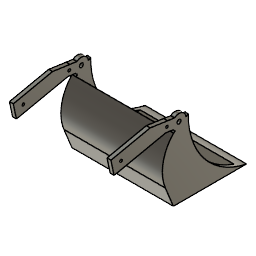
Final Scoop (Autodesk Fusion 360 design; units mm, degrees)
Autodesk Fusion 360 part; units mm, degrees
sketch "Sketch1" plane through (0, 0, 0) normal (1, 0, 0) x (0, 1, 0)
  line L0 (0, 0) -> (254, 0) construction
  line L1 (0, 0) -> (50.8, 0) construction
  line L2 (50.8, 0) -> (50.8, 107.95) construction
  line L3 (50.8, 107.95) -> (117.7014, 0) construction
  line L4 (50.8, 107.95) -> (117.6994, 215.9013) construction
  line L5 (117.7014, 0) -> (212.9514, 0) construction
  line L6 (117.7014, 0) -> (24.5328, 19.8036)
  line L7 (117.7014, 0) -> (212.9514, 0) construction
  line L8 (24.5328, 19.8036) -> (19.6811, 47.3191)
  line L9 (24.5328, 19.8036) -> (52.4728, 19.8036) construction
  arc A0 (41.91, 100.33) -> (19.6811, 47.3191) centre (72.0035, 56.545) ccw
  line L10 (41.91, 100.33) -> (64.77, 100.33) construction
  arc A1 (63.3914, 108.1486) -> (117.7014, 0) centre (155.1008, 86.4922) ccw
  circle A2 centre (50.8, 107.95) radius 2.5654
  line L11 (41.91, 100.33) -> (44.3855, 101.231)
  line L12 (60.0326, 106.9261) -> (63.3914, 108.1486)
  arc A3 (55.3791, 100.33) -> (55.4831, 100.3935) centre (50.8, 107.95) ccw
  line L13 (23.6346, 124.9202) -> (23.6308, 124.9202)
  line L14 (50.8, 107.95) -> (35.8756, 113.3608) construction
  circle A4 centre (35.8756, 113.3608) radius 1.651
  line L15 (46.5903, 116.2306) -> (38.0399, 119.3306)
  arc A5 (60.0326, 106.9261) -> (46.5903, 116.2306) centre (50.8, 107.95) ccw
  arc A6 (42.2617, 104.2911) -> (44.3855, 101.231) centre (50.8, 107.95) ccw
  circle A7 centre (-24.3224, 117.475) radius 1.651
  line L16 (-35.6254, 127.2794) -> (16.51, 127.2794)
  line L17 (38.0399, 119.3306) -> (16.51, 127.2794)
  line L18 (-35.6254, 127.2794) -> (-35.6254, 107.6706)
  line L19 (-35.6254, 107.6706) -> (33.057, 107.6706)
  line L20 (33.057, 107.6706) -> (42.2617, 104.2911)
  point P0 (0, 127)
  point P1 (50.8, 107.95)
  point P2 (-24.3224, 117.475)
  dimension "d1" = 254
  dimension "d2" = 107.95
  dimension "d3" = 127
  dimension "d4" = 127
  dimension "d8" = 95.25
  dimension "d9" = 168
  dimension "d10" = 100
  dimension "d11" = 27.94
  dimension "d14" = 20
  dimension "d15" = 22.86
  dimension "d16" = 5.1308
  dimension "d17" = 17.78
  dimension "d38" = 15.875
  dimension "d40" = 3.302
  dimension "d65" = 3.302
  dimension "d68" = 19.6088
  constraint coincident L0.start L1.start
  constraint horizontal L0
  constraint coincident L0 L1.end
  constraint perpendicular L0 L2
  constraint coincident P1 L2.end
  constraint coincident L0 L3.end
  constraint horizontal L5
  constraint horizontal L7
  constraint horizontal L9
  constraint tangent L8 A0
  constraint horizontal L10
  constraint collinear L11 L12
  constraint coincident L10 A3.start
  constraint coincident L3 A3.end
  constraint concentric A3 A5
  constraint horizontal L13
  constraint concentric A5 A6
  constraint coincident P2 A7.centre
  constraint vertical L18
  constraint perpendicular L18 L19
  measures "d1" distance of L0.start L0.end
  measures "d2" distance of L1.end P1
  measures "d3" distance of P1 L3.end
  measures "d4" distance of P1 L4.end
  measures "d8" distance of L3.end L6.end
  measures "d9" angle of L6 L7
  measures "d10" angle of L8 L9
  measures "d11" distance of L6.end L8.end
  measures "d14" angle of L10 L11
  measures "d15" distance of A0.start A1.start
  measures "d16" diameter of A2
  measures "d17" diameter of A3
  measures "d38" distance of P1 L14.end
  measures "d40" diameter of A4
  measures "d65" diameter of A7
  measures "d68" distance of L16.start L18.end
extrude "Extrude1" add sketch "Sketch1" along normal blind 5.08 contours L6 L8 A0 A1 L11 L12 L15 A5 A6 L16 L17 L18 L19 L20 | A4 | A7 makes body 1
copy_body "CopyPasteBodies1" bodies 1 makes body 2
sketch "Sketch2" plane through (5.08, 0, 0) normal (1, 0, 0) x (0, 1, 0)
  circle A0 centre (50.8, 107.95) radius 2.5654
  arc A1 (42.2617, 104.2911) -> (44.3855, 101.231) centre (50.8, 107.95) ccw
  line L0 (44.3855, 101.231) -> (41.91, 100.33)
  arc A2 (41.91, 100.33) -> (19.6811, 47.3191) centre (72.0035, 56.545) ccw
  line L1 (19.6811, 47.3191) -> (24.5328, 19.8036)
  line L2 (24.5328, 19.8036) -> (117.7014, 0)
  arc A3 (63.3914, 108.1486) -> (117.7014, 0) centre (155.1008, 86.4922) ccw
  line L3 (63.3914, 108.1486) -> (60.0326, 106.9261)
  line L4 (24.5328, 19.8036) -> (117.7014, 0)
  line L5 (25.1666, 22.785) -> (118.3351, 2.9814)
  line L6 (24.5328, 19.8036) -> (25.1666, 22.785)
  line L7 (117.7014, 0) -> (118.3351, 2.9814)
  line L8 (46.5903, 116.2306) -> (38.0399, 119.3306)
  line L9 (-35.6254, 127.2794) -> (-35.6254, 107.6706)
  line L10 (-35.6254, 107.6706) -> (33.057, 107.6706)
  line L11 (33.057, 107.6706) -> (42.2617, 104.2911)
  arc A4 (60.0326, 106.9261) -> (46.5903, 116.2306) centre (50.8, 107.95) ccw
  line L12 (38.0399, 119.3306) -> (16.51, 127.2794)
  line L13 (16.51, 127.2794) -> (-35.6254, 127.2794)
  dimension "d32" = -3.048
  constraint coincident L1.end L2.start
  constraint perpendicular L5 L6
  constraint coincident L2.end A3.end
  constraint perpendicular L5 L7
extrude "Extrude2" add sketch "Sketch2" against normal up to surface (5.08 mm away) contours L2 A3 L4 L5 L6 bodies 1 2
sketch "Sketch3" plane through (5.08, 0, 0) normal (1, 0, 0) x (0, 1, 0)
  arc A0 (63.3914, 108.1486) -> (117.7014, 0) centre (155.1008, 86.4922) ccw
  line L0 (63.3914, 108.1486) -> (60.0326, 106.9261)
  arc A1 (60.0326, 106.9261) -> (46.5903, 116.2306) centre (50.8, 107.95) ccw
  line L1 (44.3855, 101.231) -> (41.91, 100.33)
  arc A2 (41.91, 100.33) -> (19.6811, 47.3191) centre (72.0035, 56.545) ccw
  line L2 (19.6811, 47.3191) -> (24.5328, 19.8036)
  circle A3 centre (50.8, 107.95) radius 2.5654
  line L3 (19.6811, 47.3191) -> (24.5328, 19.8036)
  arc A4 (41.91, 100.33) -> (19.6811, 47.3191) centre (72.0035, 56.545) ccw
  arc A5 (43.6364, 97.8181) -> (22.6828, 47.8484) centre (72.0035, 56.545) ccw
  line L4 (22.6828, 47.8484) -> (27.5345, 20.3329)
  line L5 (24.5328, 19.8036) -> (27.5345, 20.3329)
  line L6 (43.6364, 97.8181) -> (41.91, 100.33)
  line L7 (24.5328, 19.8036) -> (117.7014, 0)
  line L8 (46.5903, 116.2306) -> (38.0399, 119.3306)
  line L9 (38.0399, 119.3306) -> (16.51, 127.2794)
  line L10 (16.51, 127.2794) -> (-35.6254, 127.2794)
  line L11 (-35.6254, 127.2794) -> (-35.6254, 107.6706)
  line L12 (-35.6254, 107.6706) -> (33.057, 107.6706)
  line L13 (33.057, 107.6706) -> (42.2617, 104.2911)
  arc A6 (42.2617, 104.2911) -> (44.3855, 101.231) centre (50.8, 107.95) ccw
  dimension "d35" = -3.048
  constraint coincident L2.end L3.end
  constraint perpendicular L4 L5
  constraint coincident L1.end A2.start
extrude "Extrude3" add sketch "Sketch3" against normal up to surface (5.08 mm away) contours A2 L2 L3 A4 A5 L4 L5 L6 bodies 1
extrude "Extrude4" add sketch "Sketch1" along normal blind 5.08 separate body contours L6 L8 A0 A1 L11 L12 L15 A5 A6 L16 L17 L18 L19 L20 | A7 makes body 3
extrude "Extrude5" cut sketch "Sketch1" along normal blind 5.08 contours A4 bodies 1
copy_body "CopyPasteBodies2" bodies 3 makes body 4
move_body "Move2" bodies 4 to x (1, 0, 0) y (0, 1, 0) z (0, 0, 1) at (127, 0, 0)
sketch "Sketch4" plane through (5.08, 0, 0) normal (1, 0, 0) x (0, 1, 0)
  circle A0 centre (35.8756, 113.3608) radius 1.651
  line L0 (24.5328, 19.8036) -> (117.7014, 0)
  arc A1 (63.3914, 108.1486) -> (117.7014, 0) centre (155.1008, 86.4922) ccw
  line L1 (63.3914, 108.1486) -> (60.0326, 106.9261)
  arc A2 (60.0326, 106.9261) -> (46.5903, 116.2306) centre (50.8, 107.95) ccw
  line L2 (46.5903, 116.2306) -> (38.0399, 119.3306)
  line L3 (44.3855, 101.231) -> (41.91, 100.33)
  arc A3 (41.91, 100.33) -> (19.6811, 47.3191) centre (72.0035, 56.545) ccw
  line L4 (19.6811, 47.3191) -> (24.5328, 19.8036)
  circle A4 centre (50.8, 107.95) radius 2.5654
  line L5 (24.5328, 19.8036) -> (117.7014, 0)
  line L6 (25.1666, 22.785) -> (118.3351, 2.9814)
  line L7 (117.7014, 0) -> (118.3351, 2.9814)
  line L8 (24.5328, 19.8036) -> (25.1666, 22.785)
  line L9 (38.0399, 119.3306) -> (16.51, 127.2794)
  line L10 (16.51, 127.2794) -> (-35.6254, 127.2794)
  line L11 (-35.6254, 127.2794) -> (-35.6254, 107.6706)
  line L12 (-35.6254, 107.6706) -> (33.057, 107.6706)
  line L13 (33.057, 107.6706) -> (42.2617, 104.2911)
  arc A5 (42.2617, 104.2911) -> (44.3855, 101.231) centre (50.8, 107.95) ccw
  dimension "d50" = -3.048
  constraint coincident L0.end A1.end
  constraint perpendicular L6 L7
  constraint coincident L0.start L4.end
  constraint perpendicular L6 L8
extrude "Extrude6" add sketch "Sketch4" along normal up to surface (121.92 mm away) contours L0 A1 L5 L6 L8 bodies 1 3 4
sketch "Sketch5" plane through (5.08, 0, 0) normal (1, 0, 0) x (0, 1, 0)
  line L0 (25.1666, 22.785) -> (107.1872, 5.351)
  arc A0 (63.3914, 108.1486) -> (107.1872, 5.351) centre (155.1008, 86.4922) ccw
  line L1 (63.3914, 108.1486) -> (60.0326, 106.9261)
  arc A1 (60.0326, 106.9261) -> (46.5903, 116.2306) centre (50.8, 107.95) ccw
  line L2 (46.5903, 116.2306) -> (38.0399, 119.3306)
  line L3 (44.3855, 101.231) -> (41.91, 100.33)
  arc A2 (41.91, 100.33) -> (19.6811, 47.3191) centre (72.0035, 56.545) ccw
  line L4 (19.6811, 47.3191) -> (24.5328, 19.8036)
  line L5 (24.5328, 19.8036) -> (25.1666, 22.785)
  circle A3 centre (35.8756, 113.3608) radius 1.651
  circle A4 centre (50.8, 107.95) radius 2.5654
  line L6 (19.6811, 47.3191) -> (24.5328, 19.8036)
  arc A5 (41.91, 100.33) -> (19.6811, 47.3191) centre (72.0035, 56.545) ccw
  arc A6 (43.6364, 97.8181) -> (22.6828, 47.8484) centre (72.0035, 56.545) ccw
  line L7 (22.6828, 47.8484) -> (27.5345, 20.3329)
  line L8 (41.91, 100.33) -> (43.6364, 97.8181)
  line L9 (24.5328, 19.8036) -> (27.5345, 20.3329)
  line L10 (38.0399, 119.3306) -> (16.51, 127.2794)
  line L11 (16.51, 127.2794) -> (-35.6254, 127.2794)
  line L12 (-35.6254, 127.2794) -> (-35.6254, 107.6706)
  line L13 (-35.6254, 107.6706) -> (33.057, 107.6706)
  line L14 (33.057, 107.6706) -> (42.2617, 104.2911)
  arc A7 (42.2617, 104.2911) -> (44.3855, 101.231) centre (50.8, 107.95) ccw
  dimension "d53" = -3.048
  constraint coincident L3.end A2.start
  constraint coincident L4.end L5.start
  constraint perpendicular L7 L9
extrude "Extrude7" add sketch "Sketch5" along normal up to surface (121.92 mm away) contours L0 A2 L4 L5 L6 A5 A6 L7 L8 bodies 1
move_body "Move3" bodies 1 to x (1, 0, 0) y (0, 0.965926, 0.258819) z (0, -0.258819, 0.965926) at (0, 27.3954, -7.4284)
move_body "Move4" bodies 1 to x (1, 0, 0) y (0, 1, 0) z (0, 0, 1) at (0, -45.9671, -17.98)
move_body "Move5" bodies 1 to x (1, 0, 0) y (0, 0.998848, -0.047978) z (0, 0.047978, 0.998848) at (0, -3.9557, -0.0998)
move_body "Move6" bodies 1 to x (1, 0, 0) y (0, 1, 0) z (0, 0, 1) at (0, 3.1541, 0.9462)
move_body "Move7" bodies 1 to x (1, 0, 0) y (0, 1, 0) z (0, 0, 1) at (0, 0, -0.9387)
move_body "Move8" bodies 1 to x (1, 0, 0) y (0, 0.999994, -0.003491) z (0, 0.003491, 0.999994) at (0, -0.2875, -0.0027)
sketch "Sketch7" plane through (132.08, 0, 0) normal (1, 0, 0) x (0, 1, 0)
  circle A0 centre (6.2003, 91.6655) radius 2.5654
  circle A1 centre (-9.5249, 93.8414) radius 1.651
  line L0 (-82.3561, 92.5264) -> (-78.2625, 73.3497)
  line L1 (-78.2625, 73.3497) -> (-11.0934, 87.6882)
  line L2 (-11.0934, 87.6882) -> (-1.386, 86.3047)
  arc A2 (-1.386, 86.3047) -> (1.3299, 83.7555) centre (6.2003, 91.6655) ccw
  line L3 (1.3299, 83.7555) -> (-0.903, 82.3575)
  arc A3 (-0.903, 82.3575) -> (-11.5753, 25.8741) centre (37.6682, 45.8197) ccw
  line L4 (-11.5753, 25.8741) -> (-1.0862, -0.0223)
  line L5 (-1.0862, -0.0223) -> (94.1638, 0.0608)
  arc A4 (18.4728, 94.4884) -> (94.1638, 0.0608) centre (112.6825, 92.4549) ccw
  line L6 (18.4728, 94.4884) -> (15.4433, 92.5916)
  arc A5 (15.4433, 92.5916) -> (0.3547, 98.8849) centre (6.2003, 91.6655) ccw
  line L7 (0.3547, 98.8849) -> (-8.6545, 100.1314)
  line L8 (-8.6545, 100.1314) -> (-31.3695, 103.4105)
  line L9 (-31.3695, 103.4105) -> (-82.3561, 92.5264)
  line L10 (-80.3093, 82.938) -> (-69.0063, 82.938) construction
  circle A6 centre (-69.2533, 85.288) radius 1.651
  dimension "d70" = 11.303
  dimension "d71" = 3.302
  constraint midpoint L0 L10.start
  constraint horizontal L10
  measures "d70" distance of L10.start A6.centre
  measures "d71" diameter of A6
extrude "Extrude8" cut sketch "Sketch7" against normal blind 254 contours A6 bodies 1
